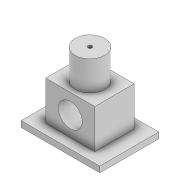
# Autodesk Inventor part: Arm_clip_template
Saved by Autodesk Inventor 2022 (Build 260153000, 153)
## iProperties
Created: 2022-08-10
Part Number: Arm_clip_template
Material: Generic
Document SubType Name: Modeling
Designer: dell
Density: 1 g/cm^3
Appearance: Default
Author: dell
Autodesk Inventor part; units mm, degrees
ref_plane "YZ Plane" through (0, 0, 0) normal (1, 0, 0) x (0, 1, 0)
ref_plane "XZ Plane" through (0, 0, 0) normal (0, 1, 0) x (-1, 0, 0)
ref_plane "XY Plane" through (0, 0, 0) normal (0, 0, 1) x (1, 0, 0)
sketch "Sketch1" plane through (0, 0, 0) normal (0, 0, 1) x (1, 0, 0)
  circle A0 centre (0, 0) radius 6.05
  line L0 (-12.5, -10) -> (12.5, -10)
  line L1 (12.5, -10) -> (12.5, 10)
  line L2 (12.5, 10) -> (-12.5, 10)
  line L3 (-12.5, 10) -> (-12.5, -10)
  line L4 (-12.5, -10) -> (12.5, 10) construction
  line L5 (12.5, -10) -> (-12.5, 10) construction
  dimension "d0" = 12.1
  dimension "d1" = 25
  dimension "d2" = 20
  constraints: 12 end point, 2 midpoint, 2 parallel, 1 centre point, 1 coincident, 1 horizontal, 1 perpendicular
  measures "d0" diameter of A0
  measures "d1" distance between parallel lines of L3 L1
  measures "d2" distance between parallel lines of L2 L0
extrude "Extrusion1" add sketch "Sketch1" along normal blind 20
sketch "Sketch2" plane through (-12.5, 10, 0) normal (0, 1, 0) x (1, 0, 0)
  line L0 (0, 0) -> (0, -20) construction
  line L1 (25, -20) -> (0, -20) construction
  line L2 (0, 0) -> (25, -20) construction
  line L3 (0, -20) -> (25, 0) construction
  circle A0 centre (12.5, -10) radius 1
  point P0 (12.5, 0)
  dimension "d5" = 2
  constraints: 4 end point, 1 centre point, 1 midpoint
  measures "d5" diameter of A0
extrude "Extrusion2" cut sketch "Sketch2" against normal blind 100
sketch "Sketch3" plane through (-12.5, 10, 0) normal (0, 1, 0) x (1, 0, 0)
  circle A0 centre (12.5, -10) radius 1 projected
  line L0 (25, 0) -> (0, 0) projected
  line L1 (0, 0) -> (0, -20) projected
  line L2 (25, -20) -> (0, -20) projected
  line L3 (25, 0) -> (25, -20) projected
  circle A1 centre (12.5, -10) radius 7.5
  point P0 (12.5, 0)
  dimension "d8" = 15
  constraints: 1 centre point, 1 coincident
  measures "d8" diameter of A1
extrude "Extrusion3" add sketch "Sketch3" along normal blind 15 contours A1
sketch "Sketch4" plane through (-12.5, -10, 0) normal (0, -1, 0) x (1, 0, 0)
  line L0 (32.5, 25) -> (-7.5, 25)
  line L1 (-7.5, 25) -> (-7.5, -5)
  line L2 (-7.5, -5) -> (32.5, -5)
  line L3 (32.5, -5) -> (32.5, 25)
  circle A0 centre (12.5, 10) radius 1 projected
  line L4 (32.5, 25) -> (-7.5, -5) construction
  line L5 (-7.5, 25) -> (32.5, -5) construction
  point P0 (12.5, 0)
  dimension "d11" = 30
  dimension "d12" = 40
  constraints: 12 end point, 2 midpoint, 2 parallel, 1 horizontal, 1 perpendicular
  measures "d11" distance of L0.end L1.end
  measures "d12" distance of L1.end L2.end
extrude "Extrusion4" add sketch "Sketch4" along normal blind 3
body "Solid1"
